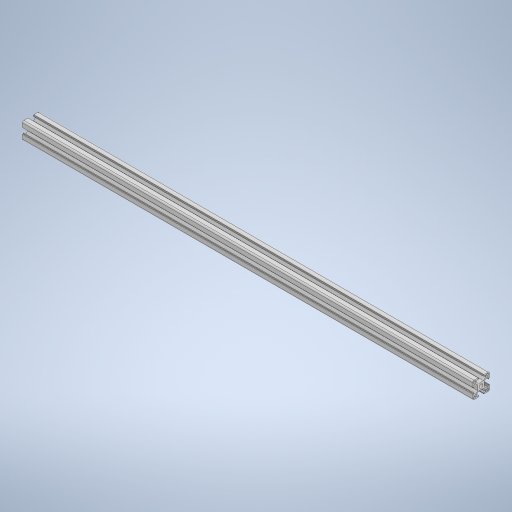
# Autodesk Inventor part: 3030_Extrusion
Saved by Autodesk Inventor 2023 (Build 270158000, 158)
## iProperties
Created: 2022-04-29
Part Number: 3030_Extrusion
Material: Generic
Document SubType Name: Modeling
Designer: plebbb
Density: 1 g/cm^3
Appearance: Default
Author: plebbb
Autodesk Inventor part; units mm, degrees
ref_plane "YZ Plane" through (0, 0, 0) normal (1, 0, 0) x (0, 1, 0)
ref_plane "XZ Plane" through (0, 0, 0) normal (0, 1, 0) x (-1, 0, 0)
ref_plane "XY Plane" through (0, 0, 0) normal (0, 0, 1) x (1, 0, 0)
sketch "Sketch1" plane through (0, 0, 0) normal (1, 0, 0) x (0, 1, 0)
  arc A0 (2.4042, 2.4042) -> (0, 3.4) centre (0, 0) ccw
  line L0 (0, 3.4) -> (0, 5.8)
  line L1 (0, 5.8) -> (4.3858, 5.8)
  line L2 (4.3858, 5.8) -> (8.25, 9.6642)
  line L3 (8.25, 9.6642) -> (8.25, 12.8)
  line L4 (8.25, 12.8) -> (4.1, 12.8)
  line L5 (4.1, 12.8) -> (4.1, 13.9)
  line L6 (4.1, 13.9) -> (5.2, 13.9)
  line L7 (5.2, 13.9) -> (5.2, 15)
  line L8 (5.2, 15) -> (12.5, 15)
  arc A1 (14.2678, 14.2678) -> (12.5, 15) centre (12.5, 12.5) ccw
  line L9 (14.2678, 14.2678) -> (13.2071, 13.2071)
  line L10 (9.75, 9.75) -> (9.75, 10.75) construction
  line L11 (10.75, 13.5) -> (12.5, 13.5)
  arc A2 (9.75, 10.75) -> (10.0429, 10.0429) centre (10.75, 10.75) ccw
  arc A3 (13.2071, 13.2071) -> (12.5, 13.5) centre (12.5, 12.5) ccw
  arc A4 (10.75, 13.5) -> (9.75, 12.5) centre (10.75, 12.5) ccw
  line L12 (12.5, 13.5) -> (13.5, 13.5) construction
  line L13 (9.75, 10.75) -> (9.75, 12.5)
  line L14 (13.2071, 13.2071) -> (10.0429, 10.0429) construction
  line L15 (10.0429, 10.0429) -> (2.4042, 2.4042)
  point P0 (8.25, 11.2321)
  dimension "d0" = 3.4
  dimension "d1" = 45
  dimension "d3" = 45
  dimension "d4" = 2.5
  dimension "d5" = 135
  dimension "d6" = 1
  dimension "d7" = 4.1
  dimension "d8" = 5.2
  dimension "d9" = 8.25
  dimension "d10" = 15
  dimension "d11" = 2.2
  dimension "d12" = 5.8
  dimension "d13" = 1.5
  dimension "d14" = 1.5
  dimension "d15" = 1
  dimension "d16" = 1
  dimension "d17" = 1
  constraints: 32 end point, 10 point on circle, 9 perpendicular, 9 point on line, 9 tangent, 5 centre point, 5 parallel, 3 vertical, 2 line through centre, 1 coincident, 1 horizontal, 1 midpoint, 1 vertical alignment
  measures "d0" radius of A0
  measures "d4" radius of A1
  measures "d5" angle of L1 L2
  measures "d6" distance between parallel lines of L9 L2
  measures "d7" horizontal distance of A0.centre L4.end
  measures "d8" horizontal distance of A0.centre L7.end
  measures "d9" distance from line of A0.centre L3
  measures "d10" distance from line of A0.centre L8
  measures "d11" distance between parallel lines of L8 L4
  measures "d12" distance from line of A0.centre L1
  measures "d13" distance from line of point (8.25, 11.232) L10
  measures "d14" distance between parallel lines of L8 L11
  measures "d15" radius of A3
  measures "d16" radius of A2
  measures "d17" radius of A4
extrude "Extrusion1" add sketch "Sketch1" along normal blind 800
mirror "Mirror1" about plane through (0, 2.4042, 2.4042) normal (0, 0.7071068, -0.7071068)
pattern_circular "Circular Pattern1" count 4 over 360 about axis through (-10, 0, 0) along (1, 0, 0)
equation "\"d18\" = LEN"
equation "\"LEN\" = 800"
body "Solid1"
